Autodesk Fusion 360 part; units mm, degrees
(part 2 of 2)
  line L717 (2.6956, 2.4051, 1.57) -> (2.6956, 1.1351, 1.57)
  line L718 (2.6956, 15.1051, 1.57) -> (2.6956, 13.8351, 1.57)
  line L719 (7.2166, 19.1849, 1.57) -> (2.9434, 19.1849, 1.57)
  line L720 (7.2166, 6.4849, 1.57) -> (2.9434, 6.4849, 1.57)
  line L721 (7.4644, 13.8351, 1.57) -> (7.4644, 15.1051, 1.57)
  line L722 (7.4644, 1.1351, 1.57) -> (7.4644, 2.4051, 1.57)
  line L723 (2.9434, 19.1849, 1.57) -> (2.9434, 17.9149, 1.57)
  line L724 (2.9434, 6.4849, 1.57) -> (2.9434, 5.2149, 1.57)
  line L725 (2.9434, 17.9149, 1.57) -> (7.2166, 17.9149, 1.57)
  line L726 (2.9434, 5.2149, 1.57) -> (7.2166, 5.2149, 1.57)
  line L727 (7.2166, 5.2149, 1.57) -> (7.2166, 6.4849, 1.57)
  line L728 (7.2166, 17.9149, 1.57) -> (7.2166, 19.1849, 1.57)
  line L729 (2.6956, 13.8351, 1.57) -> (7.4644, 13.8351, 1.57)
  line L730 (2.6956, 1.1351, 1.57) -> (7.4644, 1.1351, 1.57)
  line L731 (4.407, 16.91, 1.57) -> (4.407, 16.11, 1.57)
  line L732 (4.407, 4.21, 1.57) -> (4.407, 3.41, 1.57)
  line L733 (6.007, 16.91, 1.57) -> (4.407, 16.91, 1.57)
  line L734 (6.007, 4.21, 1.57) -> (4.407, 4.21, 1.57)
  line L735 (4.407, 16.11, 1.57) -> (6.007, 16.11, 1.57)
  line L736 (4.407, 3.41, 1.57) -> (6.007, 3.41, 1.57)
  line L737 (5.707, 16.91, 1.57) -> (5.707, 16.11, 1.57)
  line L738 (5.707, 4.21, 1.57) -> (5.707, 3.41, 1.57)
  line L739 (6.007, 4.21, 1.57) -> (4.407, 3.41, 1.57)
  line L740 (6.007, 16.91, 1.57) -> (4.407, 16.11, 1.57)
  line L741 (4.707, 4.21, 1.57) -> (4.707, 3.41, 1.57)
  line L742 (4.707, 16.91, 1.57) -> (4.707, 16.11, 1.57)
  line L743 (4.407, 4.21, 1.57) -> (6.007, 3.41, 1.57)
  line L744 (4.407, 16.91, 1.57) -> (6.007, 16.11, 1.57)
  line L745 (6.007, 16.11, 1.57) -> (6.007, 16.91, 1.57)
  line L746 (6.007, 3.41, 1.57) -> (6.007, 4.21, 1.57)
  arc A104 through (4.857, 3.81, 1.92) (5.207, 3.46, 1.92) (5.557, 3.81, 1.92)
  arc A105 through (4.857, 16.51, 1.92) (5.207, 16.16, 1.92) (5.557, 16.51, 1.92)
  line L747 (5.927, 4.17, 1.92) -> (4.487, 3.45, 1.92)
  line L748 (5.927, 16.87, 1.92) -> (4.487, 16.15, 1.92)
  line L749 (4.787, 4.17, 1.92) -> (4.787, 3.45, 1.92)
  line L750 (4.787, 16.87, 1.92) -> (4.787, 16.15, 1.92)
  line L751 (5.207, 3.81, 1.92) -> (4.857, 3.81, 1.92)
  line L752 (5.207, 16.51, 1.92) -> (4.857, 16.51, 1.92)
  line L753 (5.627, 4.17, 1.92) -> (4.787, 3.45, 1.92)
  line L754 (5.627, 16.87, 1.92) -> (4.787, 16.15, 1.92)
  line L755 (4.487, 4.17, 1.92) -> (4.487, 3.45, 1.92)
  line L756 (4.487, 16.87, 1.92) -> (4.487, 16.15, 1.92)
  line L757 (5.207, 16.51, 1.92) -> (5.557, 16.51, 1.92)
  line L758 (5.207, 3.81, 1.92) -> (5.557, 3.81, 1.92)
  line L759 (4.487, 4.17, 1.92) -> (5.927, 3.45, 1.92)
  line L760 (4.487, 16.87, 1.92) -> (5.927, 16.15, 1.92)
  line L761 (4.487, 3.45, 1.92) -> (5.927, 3.45, 1.92)
  line L762 (4.487, 16.15, 1.92) -> (5.927, 16.15, 1.92)
  line L763 (5.627, 16.87, 1.92) -> (5.627, 16.15, 1.92)
  line L764 (5.627, 4.17, 1.92) -> (5.627, 3.45, 1.92)
  line L765 (5.927, 3.45, 1.92) -> (5.927, 4.17, 1.92)
  line L766 (5.927, 16.15, 1.92) -> (5.927, 16.87, 1.92)
  line L767 (5.927, 4.17, 1.92) -> (4.487, 4.17, 1.92)
  line L768 (5.927, 16.87, 1.92) -> (4.487, 16.87, 1.92)
  line L769 (5.127, 16.55, 1.75) -> (5.127, 16.47, 1.75)
  line L770 (5.127, 3.85, 1.75) -> (5.127, 3.77, 1.75)
  line L771 (5.127, 3.85, 1.75) -> (5.287, 3.77, 1.75)
  line L772 (5.127, 16.55, 1.75) -> (5.287, 16.47, 1.75)
  line L773 (5.127, 16.47, 1.75) -> (5.287, 16.47, 1.75)
  line L774 (5.127, 3.77, 1.75) -> (5.287, 3.77, 1.75)
  line L775 (5.287, 3.77, 1.75) -> (5.287, 3.85, 1.75)
  line L776 (5.287, 16.47, 1.75) -> (5.287, 16.55, 1.75)
  line L777 (5.287, 16.55, 1.75) -> (5.127, 16.55, 1.75)
  line L778 (5.287, 3.85, 1.75) -> (5.127, 3.85, 1.75)
  line L779 (5.287, 3.85, 1.75) -> (5.127, 3.77, 1.75)
  line L780 (5.287, 16.55, 1.75) -> (5.127, 16.47, 1.75)
  point P0 (-0.7, 0)
  point P1 (0.7, 0)
  point P2 (0, -0.95)
  point P3 (0, -0.95)
  point P4 (0, 0.95)
  point P5 (0, 0.95)
  point P6 (-1.016, 0)
  point P7 (-1.016, 0)
  point P8 (5, 4.7)
  point P9 (5, 4.7)
  point P10 (7, 5.5)
  point P11 (7, 5.5)
  point P12 (1, 5.5)
  point P13 (1, 5.5)
  point P14 (7, 5.5)
  point P15 (7, 5.5)
  point P16 (0, 5.5)
  point P17 (0, 5.5)
  point P18 (1, 5.5)
  point P19 (1, 5.5)
  point P20 (0, 1)
  point P21 (0, 1)
  point P22 (0, 2.4)
  point P23 (0, 2.4)
  point P24 (0, 5)
  point P25 (0, 5)
  point P26 (0, 2)
  point P27 (0, 2)
  point P28 (0, 5.5)
  point P29 (0, 5.5)
  point P30 (0, 2.4)
  point P31 (0, 2.4)
  point P32 (0, 3.9)
  point P33 (0, 3.9)
  point P34 (0, 5.5)
  point P35 (0, 5.5)
  point P36 (8, 3.9)
  point P37 (8, 3.9)
  point P38 (8, 0)
  point P39 (8, 0)
  point P40 (8, 0)
  point P41 (8, 0)
  point P42 (8, 2.4)
  point P43 (8, 2.4)
  point P44 (8, 0)
  point P45 (8, 0)
  point P46 (8, 1)
  point P47 (8, 1)
  point P48 (0, 0.5703)
  point P49 (0, 0.5703)
  point P50 (0, 4)
  point P51 (0, 4)
  point P52 (5, 3)
  point P53 (5, 3)
  point P54 (3, 3)
  point P55 (3, 3)
  point P56 (4, 5.5)
  point P57 (4, 5.5)
  point P58 (6, 5.5)
  point P59 (6, 5.5)
  point P60 (2, 5.5)
  point P61 (2, 5.5)
  point P62 (0, 5)
  point P63 (0, 5)
  point P64 (2.5, 5)
  point P65 (2.5, 5)
  point P66 (5.5, 5)
  point P67 (5.5, 5)
  point P68 (0, 5)
  point P69 (0, 5)
  point P70 (0, -0.95)
  point P71 (0, 0.95)
  dimension "d1" = 2.5426
  measures "d1" distance of L3 A0.centre
extrude "Extruir1" add sketch "Boceto1" against normal blind 2 from surface at 1.57
extrude "Extruir2" cut sketch "Boceto1" against normal blind 3 contours A42 L715 L717 | A42 L715 L717 | A40 L723 | A40 L723 | A41 | L279 L286 L291 L304 | L280 L285 L292 L303 | L281 L287 L296 L298 | L282 L288 L295 L297 in plane through (0, 0, 1.57) normal (0, 0, 1)
